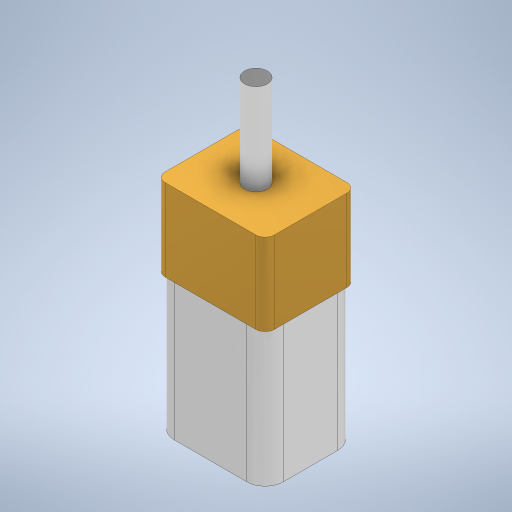
# Autodesk Inventor part: DC 6V 200RPM
Saved by Autodesk Inventor 2024 (Build 280153000, 153)
## iProperties
Created: 2023-10-18
Part Number: DC 6V 200RPM
Material: Generic
Document SubType Name: Modeling
Designer: CJ110
Density: 1 g/cm^3
Appearance: Default
Author: CJ110
Autodesk Inventor part; units mm, degrees
ref_plane "YZ Plane" through (0, 0, 0) normal (1, 0, 0) x (0, 1, 0)
ref_plane "XZ Plane" through (0, 0, 0) normal (0, 1, 0) x (-1, 0, 0)
ref_plane "XY Plane" through (0, 0, 0) normal (0, 0, 1) x (1, 0, 0)
sketch "Sketch1" plane through (0, 0, 0) normal (0, 1, 0) x (-1, 0, 0)
  line L0 (0, 0) -> (12, 0)
  line L1 (12, 0) -> (12, 10)
  line L2 (12, 10) -> (0, 10)
  line L3 (0, 10) -> (0, 0)
  dimension "d0" = 10
  dimension "d1" = 12
  constraints: 8 end point, 2 parallel, 1 horizontal, 1 perpendicular
  measures "d0" distance of L0.end L1.end
  measures "d1" distance of L1.end L2.end
extrude "Extrusion1" add sketch "Sketch1" along normal blind 15
sketch "Sketch2" plane through (0, 15, 0) normal (0, 1, 0) x (1, 0, 0)
  line L0 (-12, 0) -> (-12, -10) projected
  line L1 (-12, -10) -> (0, -10) projected
  line L2 (0, -10) -> (0, 0) projected
  line L3 (0, 0) -> (-12, 0) projected
extrude "Extrusion2" add sketch "Sketch2" along normal blind 9 separate body
sketch "Sketch3" plane through (0, 24, 0) normal (0, 1, 0) x (1, 0, 0)
  line L0 (-12, 0) -> (-12, -10) construction
  line L1 (-12, -5) -> (0, -5) construction
  line L2 (0, -10) -> (0, 0) construction
  line L3 (-12, -10) -> (0, -10) construction
  line L4 (-6, -10) -> (-6, 0) construction
  line L5 (0, 0) -> (-12, 0) construction
  circle A0 centre (-6, -5) radius 1.25
  dimension "d6" = 2.5
  constraints: 5 midpoint, 4 end point, 1 centre point
  measures "d6" diameter of A0
extrude "Extrusion3" add sketch "Sketch3" along normal blind 10 separate body
fillet "Fillet1" radius 2 4 edges at (0, 7.5, 10) (0, 7.5, 0) (-12, 7.5, 0) (-12, 7.5, 10)
fillet "Fillet2" radius 1 4 edges at (0, 19.5, 0) (-12, 19.5, 0) (0, 19.5, 10) (-12, 19.5, 10)
